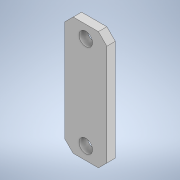
# Autodesk Inventor part: リンク26×6×2
Saved by Autodesk Inventor 2021 (Build 250183000, 183)
## iProperties
Created: 2021-10-09
Part Number: リンク26×6×2
Material: 一般
Document SubType Name: Modeling
Designer: ryusei
Density: 1 g/cm^3
Appearance: 既定
Author: ryusei
Autodesk Inventor part; units mm, degrees
ref_plane "YZ Plane" through (0, 0, 0) normal (1, 0, 0) x (0, 1, 0)
ref_plane "XZ Plane" through (0, 0, 0) normal (0, 1, 0) x (-1, 0, 0)
ref_plane "XY Plane" through (0, 0, 0) normal (0, 0, 1) x (1, 0, 0)
sketch "スケッチ1" plane through (0, 0, 0) normal (0, 0, 1) x (1, 0, 0)
  line L0 (0, 0) -> (10, 0)
  line L1 (10, 0) -> (10, 28)
  line L2 (10, 28) -> (0, 28)
  line L3 (0, 28) -> (0, 0)
  dimension "d0" = 10
  dimension "d1" = 28
  constraints: 8 end point, 2 parallel, 1 horizontal, 1 perpendicular
  measures "d0" distance of L0.start L0.end
  measures "d1" distance of L0.end L1.end
extrude "押し出し1" add sketch "スケッチ1" along normal blind 2
sketch "スケッチ2" plane through (0, 0, 2) normal (0, 0, 1) x (1, 0, 0)
  line L0 (10, 28) -> (0, 28) projected
  line L1 (10, 0) -> (10, 28) projected
  line L2 (0, 0) -> (10, 0) projected
  point P0 (5, 3)
  dimension "d6" = 5
  dimension "d7" = 3
  measures "d6" distance from line of L1 point (5, 3)
  measures "d7" distance from line of L2 point (5, 3)
hole "穴1" at (5, 3, 2) direction (0, 0, -1) diameter 3.2 end through all
sketch "スケッチ7" plane through (0, 0, 2) normal (0, 0, 1) x (1, 0, 0)
  line L0 (10, 0) -> (10, 28) projected
  line L1 (10, 28) -> (0, 28) projected
  point P0 (0, 0)
  point P1 (5, 25)
  point P2 (6, 3)
  point P3 (6, 27)
  point P4 (5, 28)
  point P5 (1, 28)
  point P6 (6, 2)
  dimension "d43" = 5
  dimension "d44" = 3
  constraints: 1 other
  measures "d44" distance from line of L1 point (5, 25)
hole "穴2" at (5, 25, 2) direction (0, 0, -1) diameter 3.2 end through all
sketch "スケッチ8" plane through (0, 0, 2) normal (0, 0, 1) x (1, 0, 0)
  line L0 (10, 28) -> (0, 28) projected
  line L1 (8, 28) -> (10, 26)
  line L2 (10, 0) -> (10, 28) projected
  line L3 (0, 28) -> (0, 0) projected
  line L4 (0, 26) -> (2, 28)
  line L5 (0, 0) -> (10, 0) projected
  line L6 (2, 0) -> (0, 2)
  line L7 (8, 0) -> (10, 2)
  dimension "d45" = 2
  dimension "d46" = 2
  dimension "d49" = 2
  dimension "d50" = 2
  dimension "d51" = 2
  dimension "d52" = 2
  dimension "d53" = 2
  dimension "d54" = 2
  constraints: 8 end point, 8 point on line
  measures "d45" horizontal distance of L1.start L1.end
  measures "d46" horizontal distance of L1.start L1.end
  measures "d49" horizontal distance of L4.start L4.end
  measures "d50" horizontal distance of L4.start L4.end
  measures "d51" horizontal distance of L6.start L6.end
  measures "d52" horizontal distance of L6.start L6.end
  measures "d53" horizontal distance of L7.start L7.end
  measures "d54" horizontal distance of L7.start L7.end
extrude "押し出し5" cut sketch "スケッチ8" against normal blind 10 contours L2 L1 L0 | L4 L3 L0 | L2 L5 L7 | L6 L5 L3
